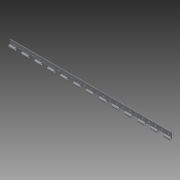
# Autodesk Inventor part: continuous hinge bottom
Saved by Autodesk Inventor 2015 SP1 (Build 190203100, 203)
## iProperties
Created: 2015-01-27
Part Number: continuous hinge bottom
Material: Generic
Document SubType Name: Modeling
Designer: Admin
Density: 1 g/cm^3
Appearance: Default
Author: Admin
Autodesk Inventor part; units mm, degrees
ref_plane "YZ Plane" through (0, 0, 0) normal (1, 0, 0) x (0, 1, 0)
ref_plane "XZ Plane" through (0, 0, 0) normal (0, 1, 0) x (-1, 0, 0)
sketch "Sketch1" plane through (0, 0, 0) normal (1, 0, 0) x (0, 1, 0)
  line L0 (0, 0) -> (25.4, 0) construction
  line L1 (25.4, 0) -> (25.4, -1.5875) construction
  line L2 (25.4, -1.5875) -> (0, -1.5875) construction
  line L3 (0, -1.5875) -> (0, 0) construction
  circle A0 centre (4.7625, 3.175) radius 4.7625 construction
  line L4 (25.4, 0) -> (25.4, -1.5875)
  line L5 (25.4, -1.5875) -> (4.7625, -1.5875)
  line L6 (25.4, 0) -> (8.3123, 0)
  arc A1 (8.3123, 0) -> (4.7625, -1.5875) centre (4.7625, 3.175) ccw
  dimension "d0" = 25.4
  dimension "d1" = 1.5875
  dimension "d2" = 9.525
  dimension "d3" = 4.7625
  dimension "d4" = 3.175
  constraints: 14 end point, 4 point on circle, 2 centre point, 2 parallel, 2 point on line, 1 horizontal, 1 perpendicular, 1 tangent, 1 vertical
  measures "d0" distance of L1.end L2.end
  measures "d1" distance of L0.end L1.end
  measures "d2" diameter of A0
  measures "d3" horizontal distance of L0.start A0.centre
  measures "d4" vertical distance of L0.start A0.centre
extrude "Extrusion1" add sketch "Sketch1" along normal blind 635
sketch "Sketch2" plane through (635, 0, 0) normal (1, 0, 0) x (0, 0, -1)
  arc A0 (0, 8.3123) -> (1.5875, 4.7625) centre (-3.175, 4.7625) ccw projected
  circle A1 centre (-3.175, 4.7625) radius 3.175
  point P0 (0, 0)
  dimension "d7" = 6.35
  constraints: 1 centre point, 1 coincident
  measures "d7" diameter of A1
extrude "Extrusion2" cut sketch "Sketch2" against normal blind 635
sketch "Sketch4" plane through (635, 25.4, -1.5875) normal (0, 0, -1) x (-1, 0, 0)
  line L0 (635, 0) -> (0, 0) projected
  line L1 (0, -20.6375) -> (0, 0) projected
  point P0 (0, -17.0877)
  point P1 (635, -25.4)
  point P2 (12.7, -9.525)
  dimension "d15" = 9.525
  dimension "d16" = 12.7
  measures "d15" distance from line of L0 point (12.7, -9.525)
  measures "d16" distance from line of L1 point (12.7, -9.525)
hole "Hole1" at (622.3, 15.875, -1.5875) direction (0, 0, 1) diameter 6.35 end through all
pattern_linear "Rectangular Pattern2" count 25 spacing 25.4 along (-1, 0, 0) of "Hole1"
ref_plane "Work Plane1" through (609.6, 0, 0) normal (1, 0, 0) x (0, 0, -1)
sketch "Sketch5" plane through (609.6, 0, 0) normal (1, 0, 0) x (0, 0, -1)
  circle A0 centre (-3.175, 4.7625) radius 3.175 projected
  line L0 (1.5875, 25.4) -> (0, 25.4) projected
  line L1 (0, 25.4) -> (0, 8.3123) projected
  arc A1 (0, 8.3123) -> (1.5875, 4.7625) centre (-3.175, 4.7625) ccw projected
  line L2 (1.5875, 4.7625) -> (1.5875, 25.4) projected
  line L3 (0, 8.3123) -> (1.5875, 8.3123)
  line L4 (1.5875, 4.7625) -> (1.5875, 25.4) projected
  line L5 (1.5875, 8.3123) -> (1.5875, 4.7625)
  arc A2 (0, 8.3123) -> (1.5875, 4.7625) centre (-3.175, 4.7625) ccw
  point P0 (0, 0)
  constraints: 4 end point, 2 point on circle, 1 centre point, 1 concentric, 1 perpendicular, 1 point on line, 1 vertical
extrude "Extrusion4" cut sketch "Sketch5" against normal blind 25.4 contours L2 A1 L3
pattern_linear "Rectangular Pattern3" count 12 spacing 50.8 along (-1, 0, 0) of "Extrusion4"
body "Solid1"
